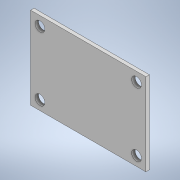
# Autodesk Inventor part: board
Saved by Autodesk Inventor 2022 (Build 260153000, 153)
## iProperties
Created: 2024-02-02
Part Number: board
Material: Generic
Document SubType Name: Modeling
Designer: Paul
Density: 1 g/cm^3
Appearance: Default
Author: Paul
Autodesk Inventor part; units mm, degrees
ref_plane "YZ Plane" through (0, 0, 0) normal (1, 0, 0) x (0, 1, 0)
ref_plane "XZ Plane" through (0, 0, 0) normal (0, 1, 0) x (-1, 0, 0)
ref_plane "XY Plane" through (0, 0, 0) normal (0, 0, 1) x (1, 0, 0)
sketch "Sketch1" plane through (0, 0, 0) normal (0, 0, 1) x (1, 0, 0)
  line L0 (0, 0) -> (53.34, 0)
  line L1 (53.34, 0) -> (53.34, 38.1)
  line L2 (53.34, 38.1) -> (0, 38.1)
  line L3 (0, 38.1) -> (0, 0)
  dimension "d0" = 53.34
  dimension "d1" = 38.1
  constraints: 8 end point, 2 parallel, 1 horizontal, 1 perpendicular
  measures "d0" distance of L1.end L2.end
  measures "d1" distance of L2.end L0.start
extrude "Extrusion1" add sketch "Sketch1" along normal blind 1.6
sketch "Sketch2" plane through (0, 0, 1.6) normal (0, 0, 1) x (1, 0, 0)
  line L0 (53.34, 38.1) -> (0, 38.1) projected
  line L1 (0, 0) -> (53.34, 0) projected
  line L2 (0, 38.1) -> (0, 0) projected
  line L3 (53.34, 0) -> (53.34, 38.1) projected
  point P0 (4.318, 33.782)
  point P1 (49.022, 33.782)
  point P2 (49.022, 4.318)
  point P3 (4.318, 4.318)
  dimension "d4" = 29.464
  dimension "d5" = 4.318
  dimension "d6" = 38.1
  dimension "d7" = 53.34
  dimension "d8" = 4.318
  dimension "d9" = 4.318
  constraints: 2 horizontal alignment, 2 vertical alignment
  measures "d4" distance of point (49.022, 4.318) point (49.022, 33.782)
  measures "d5" distance from line of L0 point (49.022, 33.782)
  measures "d6" distance between parallel lines of L0 L1
  measures "d7" distance between parallel lines of L2 L3
  measures "d8" distance from line of L3 point (49.022, 33.782)
  measures "d9" distance from line of L2 point (4.318, 33.782)
hole "Hole1" at (4.318, 33.782, 1.6) at (49.022, 33.782, 1.6) at (49.022, 4.318, 1.6) at (4.318, 4.318, 1.6) direction (0, 0, -1) diameter 4.572 end through all
equation "\"d5\" = -0.5 * d4 + 0.5 * d6"
equation "\"d8\" = d5"
equation "\"d9\" = d5"
body "Solid1"
